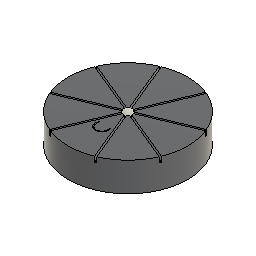
RGB_ChristmasLight_Base_v3 (Autodesk Fusion 360 design; units mm, degrees)
Autodesk Fusion 360 part; units mm, degrees
note: some values were not read from the file. Set by a fixed rule: which sketch regions a step uses.
(part 1 of 4)
sketch "Sketch1" plane through (0, 0, 0) normal (0, 0, 1) x (1, 0, 0) in component "PCB"
  circle A0 centre (0, 0) radius 30
  circle A1 centre (0, 0) radius 25 construction
  circle A2 centre (0, -25) radius 1.5
  circle A3 centre (21.6506, 12.5) radius 1.5
  circle A4 centre (-21.6506, 12.5) radius 1.5
  dimension "d1" = 60
  dimension "d2" = -5
  dimension "d3" = 3
  dimension "d5" = 360
  constraint coincident A0.centre A1.centre
  constraint coincident A1 A2.centre
  measures "d1" diameter of A0
  measures "d3" diameter of A2
extrude "Extrude1" add sketch "Sketch1" along normal blind 1.6 makes body 1 in component "PCB"
sketch "Sketch1 (2)" plane through (0, 0, 0) normal (0, 0, 1) x (1, 0, 0) in component "Enclosure_Top"
  circle A0 centre (0, 0) radius 30 construction
  circle A1 centre (0, 0) radius 32
  circle A2 centre (0, 0) radius 34
  dimension "d10" = 60
  dimension "d11" = 2
  dimension "d12" = 4
  constraint coincident A0.centre A1.centre
  measures "d10" diameter of A0
extrude "Extrude1'" add sketch "Sketch1 (2)" along normal blind 16.6 separate body contours A1 | A2 makes body 2 in component "Enclosure_Top"
extrude "Extrude2" cut sketch "Sketch1 (2)" along normal blind 12.6 contours A1 bodies 2 in component "Enclosure_Top"
sketch "Sketch2" plane through (0, 0, 1.6) normal (0, 0, 1) x (-1, 0, 0) in component "PCB"
  circle A0 centre (21.6506, -12.5) radius 1.5
  circle A1 centre (0, 25) radius 1.5
  circle A2 centre (-21.6506, -12.5) radius 1.5
  circle A3 centre (0, 0) radius 30
  circle A4 centre (0, 0) radius 2.5
  line L0 (0, 0) -> (0, 15) construction
  line L1 (0, 15) -> (6, 15) construction
  line L2 (6, 15) -> (6, 9) construction
  line L3 (6, 9) -> (-6, 9)
  line L4 (-6, 9) -> (-6, 21)
  line L5 (-6, 21) -> (6, 21)
  line L6 (6, 21) -> (6, 9)
  circle A5 centre (0, 15) radius 3.4
  dimension "d17" = 5
  dimension "d22" = 15
  dimension "d23" = 6
  dimension "d24" = 6
  dimension "d25" = 12
  dimension "d26" = 12
  dimension "d27" = 6.8
  constraint concentric A3 A4
  constraint coincident A3.centre A4.centre
  constraint vertical L0
  constraint perpendicular L0 L1
  constraint perpendicular L1 L2
  constraint horizontal L3
  constraint vertical L4
  constraint horizontal L5
  constraint vertical L6
  constraint coincident L0.end L1.start
  measures "d17" diameter of A4
  measures "d22" distance of A3.centre L0.end
  measures "d23" distance of L0.end L1.end
  measures "d24" distance of L1.end L2.end
  measures "d25" distance of L2.end L3.end
  measures "d26" distance of L2.end L5.end
  measures "d27" diameter of A5
extrude "Extrude2'" add sketch "Sketch2" along normal blind 9 contours A4 bodies 1 in component "PCB"
fillet "Fillet1" radius 2.5 1 faces at (0.8863, -0.2321, 10.6) on bodies 1 in component "PCB"
extrude "Extrude3" add sketch "Sketch2" along normal blind 7 contours A5 bodies 1 in component "PCB"
extrude "Extrude4" add sketch "Sketch2" along normal blind 3 contours L3 L4 L5 L6 bodies 1 in component "PCB"
chamfer "Chamfer1" distance 1 angle 45 4 edges at (6, -21, 3.1) (6, -9, 3.1) (-6, -9, 3.1) (-6, -21, 3.1) on bodies 1 in component "PCB"
fillet "Fillet2" radius 0.25 1 edges at (3.1699, -13.7705, 8.6) on bodies 1 in component "PCB"
sketch "Sketch2 (2)" plane through (0, 0, 16.6) normal (0, 0, 1) x (-1, 0, 0) in component "Enclosure_Top"
  circle A0 centre (0, 0) radius 34
  circle A1 centre (0, 0) radius 2.75
  line L0 (0, 0) -> (0, 15) construction
  circle A2 centre (0, 15) radius 3.65
  line L1 (0, 0) -> (-13.0112, 31.4119) construction
  line L2 (0, 0) -> (34, 0) construction
  line L3 (0.4619, 0.1913) -> (-12.5493, 31.6032)
  line L4 (-0.4619, -0.1913) -> (-13.4732, 31.2206)
  line L5 (0.5729, 2.6897) -> (12.5493, 31.6032)
  line L6 (1.4968, 2.307) -> (13.4732, 31.2206)
  line L7 (2.307, 1.4968) -> (31.2206, 13.4732)
  line L8 (2.6897, 0.5729) -> (31.6032, 12.5493)
  line L9 (2.6897, -0.5729) -> (31.6032, -12.5493)
  line L10 (2.307, -1.4968) -> (31.2206, -13.4732)
  line L11 (1.4968, -2.307) -> (13.4732, -31.2206)
  line L12 (0.5729, -2.6897) -> (12.5493, -31.6032)
  line L13 (-0.5729, -2.6897) -> (-12.5493, -31.6032)
  line L14 (-1.4968, -2.307) -> (-13.4732, -31.2206)
  line L15 (-2.307, -1.4968) -> (-31.2206, -13.4732)
  line L16 (-2.6897, -0.5729) -> (-31.6032, -12.5493)
  line L17 (-2.6897, 0.5729) -> (-31.6032, 12.5493)
  line L18 (-2.307, 1.4968) -> (-31.2206, 13.4732)
  circle A3 centre (0, 15) radius 3.15
  line L19 (3.1499, 14.9727) -> (3.1339, 13.1289)
  line L20 (-3.15, 15) -> (-3.15, 13.1561)
  dimension "d35" = 5.5
  dimension "d38" = 15
  dimension "d39" = 7.3
  dimension "d42" = 112.5
  dimension "d43" = 34
  dimension "d50" = 0.5
  dimension "d51" = -0.5
  dimension "d96" = -0.5
  constraint coincident A0.centre A1.centre
  constraint vertical L0
  constraint coincident L0.end A2.centre
  constraint horizontal L2
  constraint coincident A1 L5.start
  constraint coincident A1 L6.start
  constraint coincident A1 L7.start
  constraint coincident A1 L8.start
  constraint coincident A1 L9.start
  constraint coincident A1 L10.start
  constraint coincident A1 L11.start
  constraint coincident A1 L12.start
  constraint coincident A1 L13.start
  constraint coincident A1 L14.start
  constraint coincident A1 L15.start
  constraint coincident A1 L16.start
  constraint coincident A1 L17.start
  constraint coincident A1 L18.start
  constraint coincident A3 L19.start
  constraint coincident A2 L19.end
  constraint tangent A3 L19
  constraint coincident A3 L20.start
  constraint coincident A2 L20.end
  constraint tangent A3 L20
  constraint parallel L0 L20
  measures "d35" diameter of A1
  measures "d38" distance of A0.centre L0.end
  measures "d39" diameter of A2
  measures "d42" angle of L1 L2
  measures "d43" distance of A0.centre L1.end
extrude "Extrude3'" cut sketch "Sketch2 (2)" against normal blind 4 contours A1 bodies 2 in component "Enclosure_Top"
extrude "Extrude4'" cut sketch "Sketch2 (2)" against normal blind 4 contours A2 A3 L19 L20 | A2 A3 L19 L20 | A3 bodies 2 in component "Enclosure_Top"
extrude "Extrude6" cut sketch "Sketch2 (2)" against normal blind 3 contours A0 A1 L7 L8 | A0 A1 L9 L10 | A0 A1 L5 L6 | A0 A1 L11 L12 | A0 A1 L3 L4 | A0 A1 L13 L14 | A0 A1 L17 L18 | A0 A1 L15 L16 bodies 2 in component "Enclosure_Top"
sketch "Sketch1 (3)" plane through (0, 0, 0) normal (0, 0, 1) x (1, 0, 0) in component "Enclosure_Bottom"
  circle A0 centre (0, 0) radius 31.5
  circle A1 centre (0, 0) radius 30 construction
  circle A2 centre (0, 0) radius 25 construction
  circle A3 centre (0, -25) radius 1.75
  circle A4 centre (21.6506, 12.5) radius 1.75
  circle A5 centre (-21.6506, 12.5) radius 1.75
  line L0 (-30, 0) -> (-20.5, 0) construction
  line L1 (-20.5, 0) -> (-19.25, 0) construction
  line L2 (-19.25, 0) -> (-19.25, 2.25) construction
  line L3 (-19.25, 2.25) -> (-20.5, 2.25) construction
  line L4 (-20.5, 2.25) -> (-20.5, 0) construction
  line L5 (-19.25, 2.25) -> (-21.75, 2.25)
  line L6 (-21.75, 2.25) -> (-21.75, -2.25)
  line L7 (-21.75, -2.25) -> (-19.25, -2.25)
  line L8 (-19.25, -2.25) -> (-19.25, 2.25)
  dimension "d1_1" = 63
  dimension "d84" = 60
  dimension "d85" = -5
  dimension "d86" = 3.5
  dimension "d88" = 360
  dimension "d89" = 9.5
  dimension "d90" = 1.25
  dimension "d91" = 2.25
  dimension "d92" = 2.5
  dimension "d93" = 4.5
  constraint coincident A0.centre A1.centre
  constraint coincident A2 A3.centre
  constraint coincident A1 L0.start
  constraint horizontal L0
  constraint horizontal L1
  constraint vertical L2
  constraint horizontal L3
  constraint vertical L4
  constraint horizontal L5
  constraint vertical L6
  constraint horizontal L7
  constraint vertical L8
  measures "d1_1" diameter of A0
  measures "d84" diameter of A1
  measures "d86" diameter of A3
  measures "d89" distance of L0.start L0.end
  measures "d90" distance of L0.end L1.end
  measures "d91" distance of L0.end L3.end
  measures "d92" distance of L2.end L5.end
  measures "d93" distance of L2.end L7.end
extrude "Extrude1''" add sketch "Sketch1 (3)" along normal blind 2 separate body contours A0 | A3 | A4 | A5 | L5 L6 L7 L8 makes body 3 in component "Enclosure_Bottom"
sketch "Sketch3" plane through (0, 0, 0) normal (0, 0, -1) x (1, 0, 0) in component "PCB"
  circle A0 centre (-21.6506, -12.5) radius 1.5
  circle A1 centre (0, 25) radius 1.5
  circle A2 centre (21.6506, -12.5) radius 1.5
  circle A3 centre (0, 0) radius 30
  line L0 (-30, 0) -> (-20.5, 0) construction
  line L1 (-20.5, 0) -> (-18.3, 0) construction
  line L2 (-18.3, 0) -> (-18.3, -4.3) construction
  line L3 (-18.3, -4.3) -> (-22.7, -4.3)
  line L4 (-22.7, -4.3) -> (-22.7, 4.3)
  line L5 (-22.7, 4.3) -> (-18.3, 4.3)
  line L6 (-18.3, 4.3) -> (-18.3, -4.3)
  line L7 (-20.5, 0) -> (-21.5, 0) construction
  line L8 (-21.5, 0) -> (-21.5, -2) construction
  line L9 (-21.5, -2) -> (-20.5, -2) construction
  line L10 (-20.5, -2) -> (-20.5, 0) construction
  line L11 (-21.5, -2) -> (-19.5, -2)
  line L12 (-19.5, -2) -> (-19.5, 2)
  line L13 (-19.5, 2) -> (-21.5, 2)
  line L14 (-21.5, 2) -> (-21.5, -2)
  line L15 (0, 0) -> (0, -15) construction
  line L16 (0, -15) -> (14.275, -15) construction
  line L17 (14.275, -15) -> (14.275, -23) construction
  line L18 (14.275, -23) -> (0, -23) construction
  line L19 (0, -23) -> (0, -15) construction
  line L20 (14.275, -23) -> (-14.275, -23)
  line L21 (-14.275, -23) -> (-14.275, -7)
  line L22 (-14.275, -7) -> (14.275, -7)
  line L23 (14.275, -7) -> (14.275, -23)
  arc A4 (7.5498, -23) -> (7.5498, -7) centre (0, -15) ccw
  arc A5 (-7.5498, -7) -> (-7.5498, -23) centre (0, -15) ccw
  line L24 (14.275, -15) -> (14.275, -18.5) construction
  line L25 (14.275, -15) -> (14.275, -11.5) construction
  line L26 (14.275, -18.5) -> (10.4283, -18.5)
  line L27 (14.275, -11.5) -> (10.4283, -11.5)
  line L28 (0, -15) -> (-14.275, -15) construction
  line L29 (-14.275, -15) -> (-14.275, -18.5) construction
  line L30 (-14.275, -15) -> (-14.275, -11.5) construction
  line L31 (-14.275, -18.5) -> (-10.4283, -18.5)
  line L32 (-14.275, -11.5) -> (-10.4283, -11.5)
  circle A6 centre (0, -15) radius 10
  dimension "d56" = 9.5
  dimension "d57" = 2.2
  dimension "d58" = 4.3
  dimension "d59" = 4.4
  dimension "d60" = 8.6
  dimension "d61" = 1
  dimension "d62" = 2
  dimension "d63" = 2
  dimension "d64" = 4
  dimension "d71" = 15
  dimension "d72" = 14.275
  dimension "d73" = 8
  dimension "d74" = 28.55
  dimension "d75" = 16
  dimension "d76" = 22
  dimension "d77" = 3.5
  dimension "d78" = 3.5
  dimension "d79" = 3.5
  dimension "d80" = 3.5
  dimension "d81" = 20
  constraint coincident A3 L0.start
  constraint horizontal L0
  constraint parallel L0 L1
  constraint perpendicular L1 L2
  constraint horizontal L3
  constraint vertical L4
  constraint horizontal L5
  constraint vertical L6
  constraint horizontal L7
  constraint vertical L8
  constraint horizontal L9
  constraint vertical L10
  constraint horizontal L11
  constraint vertical L12
  constraint horizontal L13
  constraint vertical L14
  constraint coincident A3.centre L15.start
  constraint vertical L15
  constraint horizontal L16
  constraint vertical L17
  constraint horizontal L18
  constraint vertical L19
  constraint horizontal L20
  constraint vertical L21
  constraint horizontal L22
  constraint vertical L23
  constraint coincident L15.end L16.start
  constraint coincident L20 A5.end
  constraint coincident L18 A4.start
  constraint coincident L22 A4.end
  constraint concentric A4 A5
  constraint coincident L22 A5.start
  constraint coincident L23 L24.end
  constraint perpendicular L16 L25
  constraint coincident A4 L26.end
  constraint perpendicular L23 L26
  constraint coincident A4 L27.end
  constraint perpendicular L23 L27
  constraint midpoint L21 L28.end
  constraint perpendicular L28 L29
  constraint perpendicular L28 L30
  constraint coincident A5 L31.end
  constraint perpendicular L29 L31
  constraint coincident A5 L32.end
  constraint perpendicular L21 L32
  constraint concentric A4 A6
  measures "d56" distance of L0.start L0.end
  measures "d57" distance of L0.end L1.end
  measures "d58" distance of L1.end L2.end
  measures "d59" distance of L2.end L3.end
  measures "d60" distance of L2.end L5.end
  measures "d61" distance of L0.end L7.end
  measures "d62" distance of L0.end L9.end
  measures "d63" distance of L8.end L11.end
  measures "d64" distance of L8.end L13.end
  measures "d71" distance of A3.centre L15.end
  measures "d72" distance of L15.end L16.end
  measures "d73" distance of L15.end L18.end
  measures "d74" distance of L17.end L20.end
  measures "d75" distance of L17.end L22.end
  measures "d76" diameter of A4
  measures "d77" distance of L16.end L24.end
  measures "d78" distance of L16.end L25.end
  measures "d79" distance of L28.end L29.end
  measures "d80" distance of L28.end L30.end
  measures "d81" diameter of A6
extrude "Extrude5" add sketch "Sketch3" along normal blind 8.7 contours L11 L12 L13 L14 bodies 1 in component "PCB"
extrude "Extrude6'" add sketch "Sketch3" along normal blind 4.7 contours L3 L4 L5 L6 bodies 1 in component "PCB"
fillet "Fillet3" radius 0.25 8 edges at (-18.3, 4.3, -2.35) (-18.3, 0, -4.7) (-20.5, 4.3, -4.7) (-22.7, 4.3, -2.35) (-22.7, -4.3, -2.35) (-20.5, -4.3, -4.7) (-22.7, 0, -4.7) (-18.3, -4.3, -2.35) on bodies 1 in component "PCB"
extrude "Extrude7" add sketch "Sketch3" along normal blind 5.3 contours L20 L22 A4 A6 | L23 A4 L26 L27 | L20 A6 | L20 L22 A6 | L20 L22 A5 A6 | L22 A6 | L21 A5 L31 L32 bodies 1 in component "PCB"
extrude "Extrude5'" cut sketch "Sketch1 (3)" along normal blind 2 contours A3 | A4 | A5 | L5 L6 L7 L8 bodies 3 in component "Enclosure_Bottom"
extrude "Extrude7'" add sketch "Sketch2 (2)" against normal blind 0.5 contours A2 A3 L19 L20 | A3 picked at (0.2428, 11.5318) bodies 2 in component "Enclosure_Top"
sketch "Sketch3 (2)" plane through (0, 0, 12.6) normal (0, 0, -1) x (1, 0, 0) in component "Enclosure_Top"
  circle A0 centre (0, 15) radius 3.65
  circle A1 centre (0, 0) radius 2.75
  circle A2 centre (0, 0) radius 32
  circle A3 centre (0, 0) radius 25 construction
  line L0 (0, 0) -> (0, 25) construction
  line L1 (0, 25) -> (0, 22) construction
  circle A4 centre (0, 25) radius 1.6
  arc A5 (0, 22) -> (2.1213, 22.8787) centre (0, 25) ccw
  line L2 (2.1213, 22.8787) -> (9.7281, 30.4855)
  line L3 (2.1213, 22.8787) -> (12.8789, 22.8787) construction
  line L4 (-2.1213, 22.8787) -> (-9.7281, 30.4855)
  arc A6 (-2.1213, 22.8787) -> (0, 22) centre (0, 25) ccw
  circle A7 centre (-21.6506, -12.5) radius 1.6
  line L5 (-20.8742, -9.6022) -> (-31.2652, -6.8179)
  arc A8 (-19.0526, -11) -> (-20.8742, -9.6022) centre (-21.6506, -12.5) ccw
  arc A9 (-18.7529, -13.2765) -> (-19.0526, -11) centre (-21.6506, -12.5) ccw
  line L6 (-18.7529, -13.2765) -> (-21.5371, -23.6675)
  circle A10 centre (21.6506, -12.5) radius 1.6
  line L7 (18.7529, -13.2765) -> (21.5371, -23.6675)
  arc A11 (19.0526, -11) -> (18.7529, -13.2765) centre (21.6506, -12.5) ccw
  arc A12 (20.8742, -9.6022) -> (19.0526, -11) centre (21.6506, -12.5) ccw
  line L8 (20.8742, -9.6022) -> (31.2652, -6.8179)
  dimension "d99" = -7
  dimension "d100" = 3
  dimension "d101" = 3.2
  dimension "d102" = 45
  dimension "d104" = 360
  constraint coincident A1.centre A2.centre
  constraint coincident A3 L0.end
  constraint vertical L0
  constraint parallel L0 L1
  constraint coincident L0.end L1.start
  constraint horizontal L3
  constraint coincident A2 L2.end
  constraint tangent A5 L2
  constraint symmetric A5.start L1 A6.end
  constraint symmetric L1 A5.end L4.start
  constraint symmetric L1 A5 A6
  constraint symmetric L1 L2.end L4.end
  measures "d100" distance of L0.end L1.end
  measures "d101" diameter of A4
  measures "d102" angle of L2 L3
extrude "Extrude8" add sketch "Sketch3 (2)" along normal blind 3.45 contours A2 A5 L2 L4 A6 | A2 L7 A11 A12 L8 | A2 L5 A8 A9 L6 bodies 2 in component "Enclosure_Top"
sketch "Sketch3 (3)" plane through (0, 0, 2) normal (0, 0, 1) x (-1, 0, 0) in component "Enclosure_Bottom"
  line L0 (19.25, 2.25) -> (21.75, 2.25)
  line L1 (21.75, 2.25) -> (21.75, -2.25)
  line L2 (21.75, -2.25) -> (19.25, -2.25)
  line L3 (19.25, -2.25) -> (19.25, 2.25)
  circle A0 centre (0, 25) radius 1.75
  circle A1 centre (21.6506, -12.5) radius 1.75
  circle A2 centre (-21.6506, -12.5) radius 1.75
  circle A3 centre (0, 0) radius 31.5
  arc A4 (2.1213, 22.8787) -> (0, 22) centre (0, 25) cw
  arc A5 (0, 22) -> (-2.1213, 22.8787) centre (0, 25) cw
  line L4 (-2.1213, 22.8787) -> (-9.3294, 30.0867)
  line L5 (2.1213, 22.8787) -> (9.3294, 30.0867)
  line L6 (-20.8742, -9.6022) -> (-30.7206, -6.9639)
  arc A6 (-20.8742, -9.6022) -> (-19.0526, -11) centre (-21.6506, -12.5) cw
  arc A7 (-19.0526, -11) -> (-18.7529, -13.2765) centre (-21.6506, -12.5) cw
  line L7 (-18.7529, -13.2765) -> (-21.3912, -23.1229)
  line L8 (18.7529, -13.2765) -> (21.3912, -23.1229)
  arc A8 (18.7529, -13.2765) -> (19.0526, -11) centre (21.6506, -12.5) cw
  arc A9 (19.0526, -11) -> (20.8742, -9.6022) centre (21.6506, -12.5) cw
  line L9 (20.8742, -9.6022) -> (30.7206, -6.9639)
  dimension "d108" = 360
extrude "Extrude6''" add sketch "Sketch3 (3)" along normal blind 5.45 contours A3 A4 A5 L4 L5 | A3 L8 A8 A9 L9 | A3 L6 A6 A7 L7 bodies 3 in component "Enclosure_Bottom"
sketch "Sketch1 (4)" plane through (0, 0, 0) normal (0, 1, 0) x (1, 0, 0) in component "_Logo v2"
  spline S0 degree 3 poles (131.3656, -14.0229) (108.294, -15.24) (86.3865, -22.7277) (67.31, -35.851) knots 0 0 0 0 1 1 1 1
  spline S1 degree 3 poles (67.31, -35.851) (54.4248, -44.741) (42.6508, -56.8325) (34.0254, -70.0352) knots 0 0 0 0 1 1 1 1
  spline S2 degree 3 poles (34.0254, -70.0352) (15.0019, -99.2188) (9.1281, -134.6994) (17.7535, -168.566) knots 0 0 0 0 1 1 1 1
  spline S3 degree 3 poles (17.7535, -168.566) (26.9875, -204.8669) (52.6256, -235.3733) (86.7833, -250.7721) knots 0 0 0 0 1 1 1 1
  spline S4 degree 3 poles (86.7833, -250.7721) (99.2188, -256.3813) (111.3367, -259.6092) (125.8094, -261.1967) knots 0 0 0 0 1 1 1 1
  spline S5 degree 3 poles (125.8094, -261.1967) (130.0692, -261.6465) (145.6267, -261.6465) (149.8865, -261.1967) knots 0 0 0 0 1 1 1 1
  spline S6 degree 3 poles (149.8865, -261.1967) (170.815, -258.8948) (188.939, -252.4919) (205.8194, -241.3794) knots 0 0 0 0 1 1 1 1
  spline S7 degree 3 poles (205.8194, -241.3794) (224.1021, -229.3673) (238.8658, -212.7779) (248.6025, -193.384) knots 0 0 0 0 1 1 1 1
  spline S8 degree 3 poles (248.6025, -193.384) (255.9579, -178.6996) (260.1383, -163.4067) (261.4348, -146.5792) knots 0 0 0 0 1 1 1 1
  spline S9 degree 3 poles (261.4348, -146.5792) (261.8317, -141.4462) (261.5935, -129.2754) (261.0379, -124.3542) knots 0 0 0 0 1 1 1 1
  spline S10 degree 3 poles (261.0379, -124.3542) (256.3813, -84.455) (233.9446, -50.1385) (199.4958, -30.2948) knots 0 0 0 0 1 1 1 1
  spline S11 degree 3 poles (199.4958, -30.2948) (179.2552, -18.6267) (154.7813, -12.7794) (131.3656, -14.0229) knots 0 0 0 0 1 1 1 1
  spline S12 degree 3 poles (149.6219, -18.9442) (185.764, -22.5954) (218.149, -42.3333) (237.9133, -72.7604) knots 0 0 0 0 1 1 1 1
  spline S13 degree 3 poles (237.9133, -72.7604) (248.2056, -88.609) (254.3704, -105.9921) (256.5665, -125.4654) knots 0 0 0 0 1 1 1 1
  spline S14 degree 3 poles (256.5665, -125.4654) (257.1221, -130.4396) (257.2015, -144.3038) (256.6988, -148.9604) knots 0 0 0 0 1 1 1 1
  spline S15 degree 3 poles (256.6988, -148.9604) (254.2117, -171.6881) (246.6181, -191.479) (233.6535, -208.8621) knots 0 0 0 0 1 1 1 1
  spline S16 degree 3 poles (233.6535, -208.8621) (214.9475, -233.9975) (187.2721, -250.825) (156.6333, -255.6933) knots 0 0 0 0 1 1 1 1
  spline S17 degree 3 poles (156.6333, -255.6933) (149.8865, -256.7517) (146.2617, -257.0163) (137.7156, -257.0163) knots 0 0 0 0 1 1 1 1
  spline S18 degree 3 poles (137.7156, -257.0163) (126.3121, -257.0163) (118.9302, -256.1431) (108.6644, -253.5767) knots 0 0 0 0 1 1 1 1
  spline S19 degree 3 poles (108.6644, -253.5767) (77.9992, -245.8773) (51.6731, -226.3246) (35.2954, -199.0196) knots 0 0 0 0 1 1 1 1
  spline S20 degree 3 poles (35.2954, -199.0196) (17.6477, -169.6508) (13.5467, -133.6146) (24.13, -101.0708) knots 0 0 0 0 1 1 1 1
  spline S21 degree 3 poles (24.13, -101.0708) (29.1042, -85.725) (37.0681, -71.6492) (47.5456, -59.5313) knots 0 0 0 0 1 1 1 1
  spline S22 degree 3 poles (47.5456, -59.5313) (51.144, -55.4038) (58.42, -48.3394) (62.4417, -45.1115) knots 0 0 0 0 1 1 1 1
  spline S23 degree 3 poles (62.4417, -45.1115) (82.259, -29.1835) (105.5952, -20.1083) (130.6777, -18.5208) knots 0 0 0 0 1 1 1 1
  spline S24 degree 3 poles (130.6777, -18.5208) (135.3608, -18.2298) (144.5948, -18.4415) (149.6219, -18.9442) knots 0 0 0 0 1 1 1 1
  spline S25 degree 3 poles (134.1438, -34.4223) (130.1485, -39.8198) (126.8413, -44.3442) (126.7883, -44.45) knots 0 0 0 0 1 1 1 1
  spline S26 degree 3 poles (126.7883, -44.45) (126.7619, -44.5558) (127.7673, -44.7146) (129.0373, -44.8204) knots 0 0 0 0 1 1 1 1
  spline S27 degree 3 poles (129.0373, -44.8204) (130.3073, -44.8998) (132.2652, -45.0585) (133.3765, -45.1379) knots 0 0 0 0 1 1 1 1
  line L0 (133.3765, -45.1379) -> (135.4138, -45.2967)
  line L1 (135.4138, -45.2967) -> (136.4985, -43.6827)
  spline S28 degree 3 poles (136.4985, -43.6827) (137.795, -41.7777) (137.1865, -41.8571) (145.3885, -42.4656) knots 0 0 0 0 1 1 1 1
  spline S29 degree 3 poles (145.3885, -42.4656) (148.299, -42.6773) (150.8125, -42.8625) (150.9713, -42.8625) knots 0 0 0 0 1 1 1 1
  spline S30 degree 3 poles (150.9713, -42.8625) (151.13, -42.8625) (151.6327, -43.6827) (152.109, -44.6617) knots 0 0 0 0 1 1 1 1
  line L2 (152.109, -44.6617) -> (152.9292, -46.4873)
  line L3 (152.9292, -46.4873) -> (157.2154, -46.7783)
  spline S31 degree 3 poles (157.2154, -46.7783) (159.5702, -46.9635) (161.5281, -47.0429) (161.581, -46.99) knots 0 0 0 0 1 1 1 1
  spline S32 degree 3 poles (161.581, -46.99) (161.6604, -46.9371) (159.041, -42.0423) (155.8131, -36.1156) knots 0 0 0 0 1 1 1 1
  spline S33 degree 3 poles (155.8131, -36.1156) (151.7121, -28.6279) (149.7542, -25.2942) (149.3838, -25.1354) knots 0 0 0 0 1 1 1 1
  spline S34 degree 3 poles (149.3838, -25.1354) (149.0663, -25.0296) (147.1348, -24.8444) (145.124, -24.7385) knots 0 0 0 0 1 1 1 1
  line L4 (145.124, -24.7385) -> (141.4198, -24.5798)
  line L5 (141.4198, -24.5798) -> (134.1438, -34.4223)
  spline S35 degree 3 poles (146.8438, -33.8667) (147.7169, -35.6129) (148.4313, -37.1475) (148.4313, -37.3063) knots 0 0 0 0 1 1 1 1
  spline S36 degree 3 poles (148.4313, -37.3063) (148.4313, -37.5708) (145.6002, -37.465) (142.4252, -37.0681) knots 0 0 0 0 1 1 1 1
  line L6 (142.4252, -37.0681) -> (141.0229, -36.9094)
  line L7 (141.0229, -36.9094) -> (143.0867, -33.8137)
  spline S37 degree 3 poles (143.0867, -33.8137) (144.1979, -32.094) (145.1504, -30.6917) (145.1769, -30.6917) knots 0 0 0 0 1 1 1 1
  spline S38 degree 3 poles (145.1769, -30.6917) (145.2298, -30.6917) (145.9706, -32.1204) (146.8438, -33.8667) knots 0 0 0 0 1 1 1 1
  spline S39 degree 3 poles (97.6313, -31.5913) (91.731, -33.7873) (86.704, -35.6923) (86.4658, -35.7981) knots 0 0 0 0 1 1 1 1
  spline S40 degree 3 poles (86.4658, -35.7981) (86.0425, -35.9569) (86.069, -36.1685) (86.8363, -38.2852) knots 0 0 0 0 1 1 1 1
  spline S41 degree 3 poles (86.8363, -38.2852) (87.286, -39.5552) (87.6829, -40.64) (87.7094, -40.6665) knots 0 0 0 0 1 1 1 1
  spline S42 degree 3 poles (87.7094, -40.6665) (87.7358, -40.7194) (90.6463, -39.661) (94.1917, -38.3646) knots 0 0 0 0 1 1 1 1
  spline S43 degree 3 poles (94.1917, -38.3646) (97.7106, -37.0417) (100.674, -36.0098) (100.7269, -36.0892) knots 0 0 0 0 1 1 1 1
  spline S44 degree 3 poles (100.7269, -36.0892) (100.8063, -36.1421) (98.769, -39.5288) (96.2025, -43.5769) knots 0 0 0 0 1 1 1 1
  line L8 (96.2025, -43.5769) -> (91.5723, -50.9587)
  line L9 (91.5723, -50.9587) -> (92.4719, -53.34)
  spline S45 degree 3 poles (92.4719, -53.34) (93.0275, -54.8481) (93.4773, -55.6683) (93.7154, -55.6154) knots 0 0 0 0 1 1 1 1
  spline S46 degree 3 poles (93.7154, -55.6154) (95.3294, -55.2185) (116.1521, -47.2281) (116.1521, -46.99) knots 0 0 0 0 1 1 1 1
  spline S47 degree 3 poles (116.1521, -46.99) (116.1521, -46.4608) (114.644, -42.7567) (114.4058, -42.6773) knots 0 0 0 0 1 1 1 1
  spline S48 degree 3 poles (114.4058, -42.6773) (114.2735, -42.6244) (111.3102, -43.6563) (107.8177, -44.9527) knots 0 0 0 0 1 1 1 1
  spline S49 degree 3 poles (107.8177, -44.9527) (104.3252, -46.2492) (101.4413, -47.281) (101.3883, -47.2546) knots 0 0 0 0 1 1 1 1
  spline S50 degree 3 poles (101.3883, -47.2546) (101.3619, -47.2017) (103.3992, -43.8679) (105.9656, -39.8198) knots 0 0 0 0 1 1 1 1
  spline S51 degree 3 poles (105.9656, -39.8198) (108.5056, -35.7452) (110.5958, -32.3056) (110.5958, -32.1204) knots 0 0 0 0 1 1 1 1
  spline S52 degree 3 poles (110.5958, -32.1204) (110.5958, -31.406) (108.9554, -27.5167) (108.6644, -27.5431) knots 0 0 0 0 1 1 1 1
  spline S53 degree 3 poles (108.6644, -27.5431) (108.4792, -27.5431) (103.5315, -29.3688) (97.6313, -31.5913) knots 0 0 0 0 1 1 1 1
  spline S54 degree 3 poles (182.4567, -33.9196) (182.1127, -34.5546) (179.7315, -38.6821) (177.1915, -43.1006) knots 0 0 0 0 1 1 1 1
  line L10 (177.1915, -43.1006) -> (172.5613, -51.1704)
  line L11 (172.5613, -51.1704) -> (176.1596, -53.2606)
  spline S55 degree 3 poles (176.1596, -53.2606) (178.144, -54.3983) (179.8902, -55.3508) (179.996, -55.3773) knots 0 0 0 0 1 1 1 1
  spline S56 degree 3 poles (179.996, -55.3773) (180.1283, -55.4038) (180.8692, -54.2925) (181.6894, -52.9167) knots 0 0 0 0 1 1 1 1
  spline S57 degree 3 poles (181.6894, -52.9167) (182.4831, -51.5408) (183.171, -50.3502) (183.224, -50.2973) knots 0 0 0 0 1 1 1 1
  spline S58 degree 3 poles (183.224, -50.2973) (183.3827, -50.165) (189.5475, -53.8692) (190.0238, -54.4248) knots 0 0 0 0 1 1 1 1
  spline S59 degree 3 poles (190.0238, -54.4248) (190.2883, -54.6894) (190.6588, -55.3773) (190.8969, -55.9065) knots 0 0 0 0 1 1 1 1
  spline S60 degree 3 poles (190.8969, -55.9065) (191.2673, -56.806) (191.2673, -57.0706) (190.8969, -58.6317) knots 0 0 0 0 1 1 1 1
  spline S61 degree 3 poles (190.8969, -58.6317) (190.2354, -61.5156) (190.0767, -61.2775) (194.0454, -63.5265) knots 0 0 0 0 1 1 1 1
  line L12 (194.0454, -63.5265) -> (197.5644, -65.5373)
  line L13 (197.5644, -65.5373) -> (198.2523, -63.3677)
  spline S62 degree 3 poles (198.2523, -63.3677) (199.099, -60.8012) (199.1519, -59.5842) (198.4375, -58.2083) knots 0 0 0 0 1 1 1 1
  spline S63 degree 3 poles (198.4375, -58.2083) (197.776, -56.9119) (197.776, -56.9383) (198.5698, -57.0706) knots 0 0 0 0 1 1 1 1
  spline S64 degree 3 poles (198.5698, -57.0706) (199.7075, -57.3087) (201.7713, -56.6208) (202.909, -55.6683) knots 0 0 0 0 1 1 1 1
  spline S65 degree 3 poles (202.909, -55.6683) (204.3113, -54.4513) (205.396, -52.2288) (205.4225, -50.456) knots 0 0 0 0 1 1 1 1
  spline S66 degree 3 poles (205.4225, -50.456) (205.4225, -48.6304) (204.6288, -46.99) (202.8031, -45.1644) knots 0 0 0 0 1 1 1 1
  spline S67 degree 3 poles (202.8031, -45.1644) (200.7923, -43.1535) (198.4904, -41.6454) (190.5, -37.0417) knots 0 0 0 0 1 1 1 1
  spline S68 degree 3 poles (190.5, -37.0417) (186.6371, -34.8192) (183.4092, -32.9671) (183.3033, -32.9142) knots 0 0 0 0 1 1 1 1
  spline S69 degree 3 poles (183.3033, -32.9142) (183.1975, -32.8348) (182.8271, -33.311) (182.4567, -33.9196) knots 0 0 0 0 1 1 1 1
  spline S70 degree 3 poles (190.8969, -43.18) (196.7971, -46.5402) (198.0671, -48.0219) (196.5325, -49.6623) knots 0 0 0 0 1 1 1 1
  spline S71 degree 3 poles (196.5325, -49.6623) (195.4742, -50.8) (193.8602, -50.3767) (189.2035, -47.7308) knots 0 0 0 0 1 1 1 1
  spline S72 degree 3 poles (189.2035, -47.7308) (187.5102, -46.7519) (186.0815, -45.9052) (186.0021, -45.8523) knots 0 0 0 0 1 1 1 1
  spline S73 degree 3 poles (186.0021, -45.8523) (185.7904, -45.6671) (187.96, -41.8042) (188.304, -41.8042) knots 0 0 0 0 1 1 1 1
  spline S74 degree 3 poles (188.304, -41.8042) (188.4098, -41.8042) (189.574, -42.4127) (190.8969, -43.18) knots 0 0 0 0 1 1 1 1
  spline S75 degree 3 poles (65.8283, -49.7946) (63.6588, -51.5144) (62.521, -52.5727) (62.6798, -52.7579) knots 0 0 0 0 1 1 1 1
  spline S76 degree 3 poles (62.6798, -52.7579) (62.7856, -52.9167) (65.7754, -56.6473) (69.2944, -61.0658) knots 0 0 0 0 1 1 1 1
  line L14 (69.2944, -61.0658) -> (75.6973, -69.0563)
  line L15 (75.6973, -69.0563) -> (79.0575, -66.3575)
  spline S77 degree 3 poles (79.0575, -66.3575) (80.9096, -64.8758) (82.4442, -63.6587) (82.4971, -63.6323) knots 0 0 0 0 1 1 1 1
  spline S78 degree 3 poles (82.4971, -63.6323) (82.6029, -63.5529) (69.4796, -47.1223) (69.3208, -47.1223) knots 0 0 0 0 1 1 1 1
  spline S79 degree 3 poles (69.3208, -47.1223) (69.2415, -47.0958) (67.6804, -48.3129) (65.8283, -49.7946) knots 0 0 0 0 1 1 1 1
  spline S80 degree 3 poles (132.424, -48.1542) (113.7179, -49.2654) (96.176, -56.0917) (81.1477, -68.0773) knots 0 0 0 0 1 1 1 1
  spline S81 degree 3 poles (81.1477, -68.0773) (77.5758, -70.9348) (70.8025, -77.7081) (67.8921, -81.3594) knots 0 0 0 0 1 1 1 1
  spline S82 degree 3 poles (67.8921, -81.3594) (57.9702, -93.7948) (51.4879, -108.4262) (49.1067, -123.6133) knots 0 0 0 0 1 1 1 1
  line L16 (49.1067, -123.6133) -> (48.7627, -125.9417)
  line L17 (48.7627, -125.9417) -> (53.4458, -125.9417)
  line L18 (53.4458, -125.9417) -> (58.1554, -125.9417)
  line L19 (58.1554, -125.9417) -> (59.7694, -123.19)
  spline S83 degree 3 poles (59.7694, -123.19) (60.6425, -121.6819) (61.5156, -120.3854) (61.7008, -120.3325) knots 0 0 0 0 1 1 1 1
  spline S84 degree 3 poles (61.7008, -120.3325) (61.886, -120.2531) (65.6431, -120.2267) (70.0352, -120.2267) knots 0 0 0 0 1 1 1 1
  line L20 (70.0352, -120.2267) -> (77.9992, -120.2531)
  line L21 (77.9992, -120.2531) -> (78.2902, -119.2742)
  spline S85 degree 3 poles (78.2902, -119.2742) (78.6077, -118.2688) (80.0365, -116.8135) (81.1477, -116.3902) knots 0 0 0 0 1 1 1 1
  spline S86 degree 3 poles (81.1477, -116.3902) (82.0738, -116.0463) (83.7406, -116.0992) (84.746, -116.5225) knots 0 0 0 0 1 1 1 1
  spline S87 degree 3 poles (84.746, -116.5225) (86.2542, -117.131) (87.8417, -119.4594) (87.8417, -121.0469) knots 0 0 0 0 1 1 1 1
  spline S88 degree 3 poles (87.8417, -121.0469) (87.8417, -121.8671) (87.1802, -123.4281) (86.4923, -124.2219) knots 0 0 0 0 1 1 1 1
  spline S89 degree 3 poles (86.4923, -124.2219) (84.164, -126.8677) (79.7454, -126.1798) (78.4225, -122.9254) knots 0 0 0 0 1 1 1 1
  line L22 (78.4225, -122.9254) -> (77.9198, -121.7083)
  line L23 (77.9198, -121.7083) -> (70.1146, -121.7083)
  line L24 (70.1146, -121.7083) -> (62.3094, -121.7083)
  line L25 (62.3094, -121.7083) -> (60.7219, -124.4335)
  line L26 (60.7219, -124.4335) -> (59.1344, -127.1323)
  line L27 (59.1344, -127.1323) -> (53.9221, -127.2117)
  spline S90 degree 3 poles (53.9221, -127.2117) (49.9269, -127.2646) (48.7098, -127.344) (48.604, -127.635) knots 0 0 0 0 1 1 1 1
  spline S91 degree 3 poles (48.604, -127.635) (48.5246, -127.8202) (48.3923, -129.196) (48.2865, -130.6513) knots 0 0 0 0 1 1 1 1
  spline S92 degree 3 poles (48.2865, -130.6513) (48.1277, -132.8473) (48.1542, -133.35) (48.4452, -133.3765) knots 0 0 0 0 1 1 1 1
  spline S93 degree 3 poles (48.4452, -133.3765) (48.6569, -133.4029) (52.6256, -133.4294) (57.2823, -133.4294) knots 0 0 0 0 1 1 1 1
  spline S94 degree 3 poles (57.2823, -133.4294) (64.5054, -133.4823) (65.7754, -133.4294) (66.0665, -133.0854) knots 0 0 0 0 1 1 1 1
  spline S95 degree 3 poles (66.0665, -133.0854) (66.2517, -132.8738) (66.9131, -131.9213) (67.5217, -130.9688) knots 0 0 0 0 1 1 1 1
  line L28 (67.5217, -130.9688) -> (68.6594, -129.249)
  line L29 (68.6594, -129.249) -> (74.9035, -129.1696)
  spline S96 degree 3 poles (74.9035, -129.1696) (82.1002, -129.0902) (81.2271, -128.7727) (83.1056, -132.2652) knots 0 0 0 0 1 1 1 1
  line L30 (83.1056, -132.2652) -> (84.3227, -134.5406)
  line L31 (84.3227, -134.5406) -> (86.9421, -134.62)
  line L32 (86.9421, -134.62) -> (89.5615, -134.6994)
  line L33 (89.5615, -134.6994) -> (90.17, -133.35)
  spline S97 degree 3 poles (90.17, -133.35) (91.6252, -130.175) (95.6469, -129.54) (98.081, -132.1065) knots 0 0 0 0 1 1 1 1
  spline S98 degree 3 poles (98.081, -132.1065) (100.1713, -134.3025) (99.8273, -137.6098) (97.3138, -139.3296) knots 0 0 0 0 1 1 1 1
  spline S99 degree 3 poles (97.3138, -139.3296) (96.3877, -139.9646) (95.9644, -140.0969) (94.5885, -140.0969) knots 0 0 0 0 1 1 1 1
  spline S100 degree 3 poles (94.5885, -140.0969) (92.419, -140.0969) (90.9373, -139.1708) (90.1435, -137.2923) knots 0 0 0 0 1 1 1 1
  line L34 (90.1435, -137.2923) -> (89.5879, -135.9958)
  line L35 (89.5879, -135.9958) -> (86.5188, -135.9958)
  line L36 (86.5188, -135.9958) -> (83.4496, -135.9958)
  line L37 (83.4496, -135.9958) -> (82.0208, -133.35)
  line L38 (82.0208, -133.35) -> (80.6185, -130.7042)
  line L39 (80.6185, -130.7042) -> (74.9829, -130.7042)
  line L40 (74.9829, -130.7042) -> (69.3738, -130.7042)
  line L41 (69.3738, -130.7042) -> (68.0244, -132.8208)
  line L42 (68.0244, -132.8208) -> (66.675, -134.9375)
  line L43 (66.675, -134.9375) -> (57.441, -134.9375)
  spline S101 degree 3 poles (57.441, -134.9375) (49.2654, -134.9375) (48.1806, -134.9904) (48.0483, -135.3608) knots 0 0 0 0 1 1 1 1
  spline S102 degree 3 poles (48.0483, -135.3608) (47.8367, -135.89) (47.8367, -138.6417) (48.0483, -140.4144) knots 0 0 0 0 1 1 1 1
  line L44 (48.0483, -140.4144) -> (48.2335, -141.8167)
  line L45 (48.2335, -141.8167) -> (58.4994, -141.8167)
  line L46 (58.4994, -141.8167) -> (68.7917, -141.8167)
  line L47 (68.7917, -141.8167) -> (69.215, -140.7583)
  spline S103 degree 3 poles (69.215, -140.7583) (70.0352, -138.7475) (72.4958, -137.3188) (74.4273, -137.7156) knots 0 0 0 0 1 1 1 1
  spline S104 degree 3 poles (74.4273, -137.7156) (78.7665, -138.6417) (80.0365, -143.8275) (76.5704, -146.4733) knots 0 0 0 0 1 1 1 1
  spline S105 degree 3 poles (76.5704, -146.4733) (75.2475, -147.4788) (73.025, -147.664) (71.4904, -146.8702) knots 0 0 0 0 1 1 1 1
  spline S106 degree 3 poles (71.4904, -146.8702) (70.3527, -146.2881) (69.0563, -144.7006) (69.0563, -143.8804) knots 0 0 0 0 1 1 1 1
  spline S107 degree 3 poles (69.0563, -143.8804) (69.0563, -143.6158) (68.8446, -143.4042) (68.6065, -143.3777) knots 0 0 0 0 1 1 1 1
  spline S108 degree 3 poles (68.6065, -143.3777) (67.9715, -143.3513) (49.5035, -143.3513) (48.7098, -143.3777) knots 0 0 0 0 1 1 1 1
  spline S109 degree 3 poles (48.7098, -143.3777) (48.1277, -143.4042) (48.1013, -143.4571) (48.26, -144.8594) knots 0 0 0 0 1 1 1 1
  spline S110 degree 3 poles (48.26, -144.8594) (48.3394, -145.6531) (48.4981, -146.976) (48.5775, -147.7698) knots 0 0 0 0 1 1 1 1
  line L48 (48.5775, -147.7698) -> (48.7363, -149.225)
  line L49 (48.7363, -149.225) -> (58.4465, -149.225)
  spline S111 degree 3 poles (58.4465, -149.225) (63.7646, -149.225) (68.2625, -149.3308) (68.4213, -149.4367) knots 0 0 0 0 1 1 1 1
  spline S112 degree 3 poles (68.4213, -149.4367) (68.58, -149.5425) (69.506, -150.786) (70.5115, -152.1883) knots 0 0 0 0 1 1 1 1
  line L50 (70.5115, -152.1883) -> (72.3106, -154.7812)
  line L51 (72.3106, -154.7813) -> (76.3588, -154.7813)
  line L52 (76.3588, -154.7813) -> (80.3804, -154.7813)
  line L53 (80.3804, -154.7813) -> (80.5656, -154.0404)
  spline S113 degree 3 poles (80.5656, -154.0404) (80.8302, -152.9556) (81.915, -151.6592) (83.0792, -151.0771) knots 0 0 0 0 1 1 1 1
  spline S114 degree 3 poles (83.0792, -151.0771) (85.5927, -149.7806) (88.6619, -151.0242) (89.826, -153.7758) knots 0 0 0 0 1 1 1 1
  spline S115 degree 3 poles (89.826, -153.7758) (90.3552, -155.0723) (90.3288, -155.9983) (89.7202, -157.2948) knots 0 0 0 0 1 1 1 1
  spline S116 degree 3 poles (89.7202, -157.2948) (87.9475, -161.1842) (82.55, -161.2635) (80.8567, -157.4006) knots 0 0 0 0 1 1 1 1
  line L54 (80.8567, -157.4006) -> (80.301, -156.1042)
  line L55 (80.301, -156.1042) -> (75.8825, -156.1042)
  line L56 (75.8825, -156.1042) -> (71.464, -156.1042)
  line L57 (71.464, -156.1042) -> (69.6648, -153.4583)
  line L58 (69.6648, -153.4583) -> (67.8656, -150.839)
  line L59 (67.8656, -150.839) -> (58.42, -150.8125)
  spline S117 degree 3 poles (58.42, -150.8125) (52.5992, -150.8125) (48.9479, -150.9183) (48.9479, -151.0506) knots 0 0 0 0 1 1 1 1
  spline S118 degree 3 poles (48.9479, -151.0506) (48.9479, -151.2094) (49.186, -152.6117) (49.5035, -154.1727) knots 0 0 0 0 1 1 1 1
  spline S119 degree 3 poles (49.5035, -154.1727) (53.0754, -172.8788) (61.7538, -188.9919) (75.4327, -202.274) knots 0 0 0 0 1 1 1 1
  spline S120 degree 3 poles (75.4327, -202.274) (96.0438, -222.2765) (124.3542, -231.0077) (153.1144, -226.1923) knots 0 0 0 0 1 1 1 1
  spline S121 degree 3 poles (153.1144, -226.1923) (166.8198, -223.9169) (180.5781, -217.9373) (191.8758, -209.3648) knots 0 0 0 0 1 1 1 1
  spline S122 degree 3 poles (191.8758, -209.3648) (209.5235, -195.9769) (221.5885, -176.7417) (225.7954, -155.3104) knots 0 0 0 0 1 1 1 1
  spline S123 degree 3 poles (225.7954, -155.3104) (226.1394, -153.4848) (226.5098, -151.5004) (226.5892, -150.8654) knots 0 0 0 0 1 1 1 1
  line L60 (226.5892, -150.8654) -> (226.7479, -149.7542)
  line L61 (226.7479, -149.7542) -> (222.0119, -149.7542)
  line L62 (222.0119, -149.7542) -> (217.2494, -149.7542)
  line L63 (217.2494, -149.7542) -> (215.6354, -152.5323)
  line L64 (215.6354, -152.5323) -> (213.995, -155.3104)
  line L65 (213.995, -155.3104) -> (205.7135, -155.3104)
  line L66 (205.7135, -155.3104) -> (197.4321, -155.3104)
  line L67 (197.4321, -155.3104) -> (197.2469, -156.1306)
  spline S124 degree 3 poles (197.2469, -156.1306) (196.85, -157.8769) (194.4423, -159.5438) (192.3521, -159.5438) knots 0 0 0 0 1 1 1 1
  spline S125 degree 3 poles (192.3521, -159.5438) (190.4735, -159.5173) (188.4363, -157.771) (187.8806, -155.7073) knots 0 0 0 0 1 1 1 1
  spline S126 degree 3 poles (187.8806, -155.7073) (186.8752, -151.8973) (191.135, -148.4577) (194.654, -150.2304) knots 0 0 0 0 1 1 1 1
  spline S127 degree 3 poles (194.654, -150.2304) (195.9504, -150.8919) (197.0881, -152.1883) (197.2998, -153.2202) knots 0 0 0 0 1 1 1 1
  line L68 (197.2998, -153.2202) -> (197.4585, -153.9875)
  line L69 (197.4585, -153.9875) -> (205.2902, -153.9875)
  line L70 (205.2902, -153.9875) -> (213.1219, -153.9875)
  line L71 (213.1219, -153.9875) -> (214.4183, -151.7121)
  spline S128 degree 3 poles (214.4183, -151.7121) (216.5615, -147.9815) (215.8735, -148.299) (221.6415, -148.246) knots 0 0 0 0 1 1 1 1
  spline S129 degree 3 poles (221.6415, -148.246) (224.3667, -148.246) (226.695, -148.1931) (226.8008, -148.1931) knots 0 0 0 0 1 1 1 1
  spline S130 degree 3 poles (226.8008, -148.1931) (226.8802, -148.1667) (227.039, -147.1348) (227.1183, -145.8383) knots 0 0 0 0 1 1 1 1
  spline S131 degree 3 poles (227.1183, -145.8383) (227.2242, -144.5683) (227.3565, -143.219) (227.4094, -142.7956) knots 0 0 0 0 1 1 1 1
  line L72 (227.4094, -142.7956) -> (227.5417, -142.0813)
  line L73 (227.5417, -142.0813) -> (218.5723, -142.0813)
  line L74 (218.5723, -142.0813) -> (209.6294, -142.0813)
  line L75 (209.6294, -142.0813) -> (208.2006, -144.2508)
  line L76 (208.2006, -144.2508) -> (206.7719, -146.4469)
  line L77 (206.7719, -146.4469) -> (200.4748, -146.5263)
  line L78 (200.4748, -146.5263) -> (194.2042, -146.5792)
  line L79 (194.2042, -146.5792) -> (193.675, -145.7325)
  spline S132 degree 3 poles (193.675, -145.7325) (193.384, -145.2563) (192.696, -143.9863) (192.1404, -142.9544) knots 0 0 0 0 1 1 1 1
  line L80 (192.1404, -142.9544) -> (191.1615, -141.0229)
  line L81 (191.1615, -141.0229) -> (188.4627, -141.0229)
  line L82 (188.4627, -141.0229) -> (185.7904, -141.0229)
  line L83 (185.7904, -141.0229) -> (185.4729, -141.9225)
  spline S133 degree 3 poles (185.4729, -141.9225) (185.129, -143.0073) (183.4092, -144.6477) (182.3773, -144.8858) knots 0 0 0 0 1 1 1 1
  spline S134 degree 3 poles (182.3773, -144.8858) (181.954, -144.9652) (181.4777, -145.0975) (181.266, -145.1504) knots 0 0 0 0 1 1 1 1
  spline S135 degree 3 poles (181.266, -145.1504) (181.0808, -145.2033) (180.4194, -145.124) (179.8108, -144.9652) knots 0 0 0 0 1 1 1 1
  spline S136 degree 3 poles (179.8108, -144.9652) (176.4242, -144.0656) (174.969, -140.4408) (176.8475, -137.5833) knots 0 0 0 0 1 1 1 1
  spline S137 degree 3 poles (176.8475, -137.5833) (178.091, -135.7048) (180.7633, -134.9375) (182.9065, -135.8371) knots 0 0 0 0 1 1 1 1
  spline S138 degree 3 poles (182.9065, -135.8371) (183.8854, -136.234) (185.1554, -137.6098) (185.5258, -138.6946) knots 0 0 0 0 1 1 1 1
  line L84 (185.5258, -138.6946) -> (185.7904, -139.409)
  line L85 (185.7904, -139.409) -> (188.8596, -139.4883)
  line L86 (188.8596, -139.4883) -> (191.9552, -139.5677)
  line L87 (191.9552, -139.5677) -> (193.4104, -142.2665)
  line L88 (193.4104, -142.2665) -> (194.8656, -144.9917)
  line L89 (194.8656, -144.9917) -> (200.4219, -144.9917)
  line L90 (200.4219, -144.9917) -> (206.0046, -144.9917)
  line L91 (206.0046, -144.9917) -> (207.3804, -142.875)
  line L92 (207.3804, -142.875) -> (208.7298, -140.7583)
  line L93 (208.7298, -140.7583) -> (218.149, -140.7583)
  line L94 (218.149, -140.7583) -> (227.5417, -140.7583)
  line L95 (227.5417, -140.7583) -> (227.5417, -137.3188)
  line L96 (227.5417, -137.3188) -> (227.5417, -133.8792)
  line L97 (227.5417, -133.8792) -> (217.0906, -133.8792)
  line L98 (217.0906, -133.8792) -> (206.666, -133.8792)
  line L99 (206.666, -133.8792) -> (206.1633, -135.0433)
  spline S139 degree 3 poles (206.1633, -135.0433) (205.8723, -135.6783) (205.1844, -136.525) (204.6288, -136.9483) knots 0 0 0 0 1 1 1 1
  spline S140 degree 3 poles (204.6288, -136.9483) (203.7556, -137.6362) (203.4381, -137.7156) (201.7448, -137.7156) knots 0 0 0 0 1 1 1 1
  spline S141 degree 3 poles (201.7448, -137.7156) (200.0779, -137.7156) (199.734, -137.6362) (198.8873, -136.9748) knots 0 0 0 0 1 1 1 1
  spline S142 degree 3 poles (198.8873, -136.9748) (196.6913, -135.3079) (196.215, -132.2388) (197.829, -130.2279) knots 0 0 0 0 1 1 1 1
  spline S143 degree 3 poles (197.829, -130.2279) (198.9931, -128.7992) (200.1573, -128.2171) (201.7448, -128.2171) knots 0 0 0 0 1 1 1 1
  spline S144 degree 3 poles (201.7448, -128.2171) (203.8615, -128.27) (205.396, -129.3019) (206.2427, -131.3127) knots 0 0 0 0 1 1 1 1
  line L100 (206.2427, -131.3127) -> (206.6396, -132.2917)
  line L101 (206.6396, -132.2917) -> (217.0113, -132.2917)
  line L102 (217.0113, -132.2917) -> (227.3565, -132.2917)
  line L103 (227.3565, -132.2917) -> (227.1713, -129.831)
  spline S145 degree 3 poles (227.1713, -129.831) (227.0654, -128.5081) (226.9331, -127.1323) (226.8273, -126.8148) knots 0 0 0 0 1 1 1 1
  line L104 (226.8273, -126.8148) -> (226.695, -126.2063)
  line L105 (226.695, -126.2063) -> (216.7467, -126.1533)
  line L106 (216.7467, -126.1533) -> (206.8248, -126.074)
  line L107 (206.8248, -126.074) -> (205.0785, -123.5604)
  line L108 (205.0785, -123.5604) -> (203.3058, -121.0469)
  line L109 (203.3058, -121.0469) -> (199.2313, -120.994)
  line L110 (199.2313, -120.994) -> (195.1302, -120.9146)
  line L111 (195.1302, -120.9146) -> (194.5746, -122.211)
  spline S146 degree 3 poles (194.5746, -122.211) (192.5373, -126.8677) (185.3671, -125.3596) (185.3671, -120.2796) knots 0 0 0 0 1 1 1 1
  spline S147 degree 3 poles (185.3671, -120.2796) (185.3671, -117.0517) (188.1188, -114.8556) (191.426, -115.4642) knots 0 0 0 0 1 1 1 1
  spline S148 degree 3 poles (191.426, -115.4642) (192.6431, -115.7023) (194.3365, -117.2104) (194.7333, -118.4275) knots 0 0 0 0 1 1 1 1
  line L112 (194.7333, -118.4275) -> (195.0508, -119.3271)
  line L113 (195.0508, -119.3271) -> (199.3106, -119.3271)
  spline S149 degree 3 poles (199.3106, -119.3271) (201.6654, -119.3271) (203.7292, -119.4329) (203.8879, -119.5387) knots 0 0 0 0 1 1 1 1
  spline S150 degree 3 poles (203.8879, -119.5387) (204.0202, -119.6446) (204.9727, -120.8881) (205.9517, -122.2904) knots 0 0 0 0 1 1 1 1
  line L114 (205.9517, -122.2904) -> (207.7244, -124.8833)
  line L115 (207.7244, -124.8833) -> (217.1171, -124.8833)
  spline S151 degree 3 poles (217.1171, -124.8833) (225.8483, -124.8833) (226.4833, -124.8569) (226.4833, -124.4071) knots 0 0 0 0 1 1 1 1
  spline S152 degree 3 poles (226.4833, -124.4071) (226.4833, -122.6079) (224.6313, -114.591) (223.1496, -110.0667) knots 0 0 0 0 1 1 1 1
  spline S153 degree 3 poles (223.1496, -110.0667) (216.6408, -89.8525) (202.5385, -72.046) (184.3617, -61.0394) knots 0 0 0 0 1 1 1 1
  spline S154 degree 3 poles (184.3617, -61.0394) (168.8042, -51.6202) (150.5744, -47.0958) (132.424, -48.1542) knots 0 0 0 0 1 1 1 1
  spline S155 degree 3 poles (142.24, -80.1158) (142.8485, -80.4333) (143.6423, -81.0419) (144.0127, -81.4917) knots 0 0 0 0 1 1 1 1
  spline S156 degree 3 poles (144.0127, -81.4917) (144.8858, -82.5235) (145.7854, -85.3546) (145.7854, -87.0744) knots 0 0 0 0 1 1 1 1
  spline S157 degree 3 poles (145.7854, -87.0744) (145.7854, -87.7623) (145.9706, -88.8735) (146.1823, -89.5085) knots 0 0 0 0 1 1 1 1
  spline S158 degree 3 poles (146.1823, -89.5085) (146.5792, -90.6992) (147.0819, -93.3979) (147.2935, -95.594) knots 0 0 0 0 1 1 1 1
  spline S159 degree 3 poles (147.2935, -95.594) (147.3729, -96.4406) (147.2406, -97.4725) (146.8438, -98.7425) knots 0 0 0 0 1 1 1 1
  spline S160 degree 3 poles (146.8438, -98.7425) (145.759, -102.3673) (144.8594, -103.4785) (142.5575, -104.2723) knots 0 0 0 0 1 1 1 1
  spline S161 degree 3 poles (142.5575, -104.2723) (141.4463, -104.6427) (141.1287, -104.8544) (141.0758, -105.3571) knots 0 0 0 0 1 1 1 1
  spline S162 degree 3 poles (141.0758, -105.3571) (140.9965, -106.0979) (141.8696, -107.7383) (143.2719, -109.4581) knots 0 0 0 0 1 1 1 1
  line L116 (143.2719, -109.4581) -> (144.3302, -110.7281)
  line L117 (144.3302, -110.7281) -> (146.3146, -110.7546)
  spline S163 degree 3 poles (146.3146, -110.7546) (147.611, -110.7546) (148.9604, -110.9663) (150.2304, -111.3367) knots 0 0 0 0 1 1 1 1
  spline S164 degree 3 poles (150.2304, -111.3367) (152.4529, -112.0246) (152.5588, -111.9981) (154.2785, -110.146) knots 0 0 0 0 1 1 1 1
  spline S165 degree 3 poles (154.2785, -110.146) (156.1835, -108.1087) (156.4746, -107.5796) (156.2894, -106.2302) knots 0 0 0 0 1 1 1 1
  spline S166 degree 3 poles (156.2894, -106.2302) (156.0777, -104.7221) (154.9135, -101.9704) (154.0669, -100.965) knots 0 0 0 0 1 1 1 1
  spline S167 degree 3 poles (154.0669, -100.965) (153.2996, -100.039) (153.4054, -99.6156) (154.4108, -99.6156) knots 0 0 0 0 1 1 1 1
  spline S168 degree 3 poles (154.4108, -99.6156) (155.0723, -99.6156) (155.2575, -99.8008) (155.7867, -100.8592) knots 0 0 0 0 1 1 1 1
  spline S169 degree 3 poles (155.7867, -100.8592) (156.1835, -101.7587) (156.5275, -102.1292) (156.8979, -102.1292) knots 0 0 0 0 1 1 1 1
  spline S170 degree 3 poles (156.8979, -102.1292) (157.5065, -102.1292) (157.5065, -102.2085) (157.4271, -98.9012) knots 0 0 0 0 1 1 1 1
  spline S171 degree 3 poles (157.4271, -98.9012) (157.4006, -97.499) (157.4535, -96.229) (157.5329, -96.0702) knots 0 0 0 0 1 1 1 1
  spline S172 degree 3 poles (157.5329, -96.0702) (157.6652, -95.885) (157.9298, -95.885) (158.3531, -96.0967) knots 0 0 0 0 1 1 1 1
  spline S173 degree 3 poles (158.3531, -96.0967) (159.1204, -96.4406) (159.5438, -97.6842) (159.5438, -99.5362) knots 0 0 0 0 1 1 1 1
  spline S174 degree 3 poles (159.5438, -99.5362) (159.5438, -100.2506) (159.6496, -100.8063) (159.7554, -100.8063) knots 0 0 0 0 1 1 1 1
  spline S175 degree 3 poles (159.7554, -100.8063) (160.1788, -100.8063) (161.1048, -99.6156) (161.6075, -98.3985) knots 0 0 0 0 1 1 1 1
  spline S176 degree 3 poles (161.6075, -98.3985) (162.2425, -96.9169) (163.1156, -96.2025) (163.83, -96.5994) knots 0 0 0 0 1 1 1 1
  spline S177 degree 3 poles (163.83, -96.5994) (164.465, -96.9433) (164.4385, -97.7106) (163.6713, -98.9012) knots 0 0 0 0 1 1 1 1
  spline S178 degree 3 poles (163.6713, -98.9012) (162.9569, -100.0654) (162.5335, -101.6) (162.9569, -101.6) knots 0 0 0 0 1 1 1 1
  spline S179 degree 3 poles (162.9569, -101.6) (163.1156, -101.6) (163.6183, -101.1767) (164.0946, -100.621) knots 0 0 0 0 1 1 1 1
  spline S180 degree 3 poles (164.0946, -100.621) (166.079, -98.3985) (166.714, -97.8958) (167.5077, -97.8958) knots 0 0 0 0 1 1 1 1
  spline S181 degree 3 poles (167.5077, -97.8958) (168.8571, -97.8958) (168.5396, -98.9277) (166.4758, -101.256) knots 0 0 0 0 1 1 1 1
  spline S182 degree 3 poles (166.4758, -101.256) (165.4704, -102.3938) (164.465, -103.4785) (164.2269, -103.6902) knots 0 0 0 0 1 1 1 1
  spline S183 degree 3 poles (164.2269, -103.6902) (163.9623, -103.8754) (163.7771, -104.3252) (163.7771, -104.6427) knots 0 0 0 0 1 1 1 1
  spline S184 degree 3 poles (163.7771, -104.6427) (163.7771, -105.2248) (163.8565, -105.2513) (165.444, -105.2248) knots 0 0 0 0 1 1 1 1
  spline S185 degree 3 poles (165.444, -105.2248) (167.3225, -105.1719) (167.6929, -105.6481) (166.2906, -106.3096) knots 0 0 0 0 1 1 1 1
  spline S186 degree 3 poles (166.2906, -106.3096) (165.8673, -106.5212) (165.1529, -106.8652) (164.756, -107.0504) knots 0 0 0 0 1 1 1 1
  spline S187 degree 3 poles (164.756, -107.0504) (164.3327, -107.2621) (163.539, -107.4208) (162.9569, -107.4208) knots 0 0 0 0 1 1 1 1
  spline S188 degree 3 poles (162.9569, -107.4208) (162.1102, -107.4208) (161.6869, -107.6325) (160.4963, -108.6644) knots 0 0 0 0 1 1 1 1
  spline S189 degree 3 poles (160.4963, -108.6644) (159.6496, -109.4052) (159.041, -110.1725) (159.041, -110.49) knots 0 0 0 0 1 1 1 1